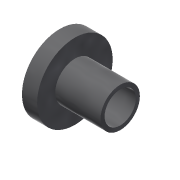
# Autodesk Inventor part: 17-0028-0031
Saved by Autodesk Inventor 2016 SP2 (Build 200236200, 236)
## iProperties
Category: IOP
Company: Universiteit van Amsterdam
Created: 2017-11-10
Part Number: 17-0028-0031
Material: Nylon Composite (Nylon, molybdenum disulphide)
Description: FJ01.1543.0390
Document SubType Name: Modeling
Designer: Daan Giesen
Density: 1.13 g/cm^3
Appearance: Textured - Gray
Mass: 0.0844545 g
Surface Area: 2.22173 cm^2
Volume: 0.0747385 cm^3
Project: Digital PID Loop
Cost Center: 17-0028
User Status: Work in Progress
Authority: Reichsöllner, Lukas
Author: Daan Giesen
Title: Digital PID Loop
Revision Number: A
Autodesk Inventor part; units mm, degrees
ref_plane "YZ Plane" through (0, 0, 0) normal (1, 0, 0) x (0, 1, 0)
ref_plane "XZ Plane" through (0, 0, 0) normal (0, 1, 0) x (-1, 0, 0)
ref_plane "XY Plane" through (0, 0, 0) normal (0, 0, 1) x (1, 0, 0)
sketch "Sketch1" plane through (0, 0, 0) normal (0, 0, 1) x (1, 0, 0)
  line L0 (0, 4.5) -> (0, -0.75) construction
  line L1 (-1.2, 0) -> (7.2, 0) construction
  line L2 (0, 3.75) -> (0, 1.55)
  line L3 (0, 1.55) -> (6, 1.55)
  line L4 (6, 1.55) -> (6, 1.95)
  line L5 (6, 1.95) -> (1.5, 1.95)
  line L6 (1.5, 1.95) -> (1.5, 3.75)
  line L7 (1.5, 3.75) -> (0, 3.75)
  point P0 (0, 0)
  dimension "d0" = 3.75
  dimension "d1" = 1.55
  dimension "d2" = 1.95
  dimension "d3" = 6
  dimension "d4" = 4.5
  constraints: 12 end point, 4 perpendicular, 2 point on line, 1 horizontal
  measures "d0" distance of point (0, 0) L2.start
  measures "d1" distance from line of point (0, 0) L3
  measures "d2" distance from line of point (0, 0) L5
  measures "d3" distance of L2.end L3.end
  measures "d4" distance of L4.end L5.end
revolve "Revolution1" add sketch "Sketch1" angle 360 about axis through (0, 0, 0) along (1, 0, 0)
body "Solid1"
